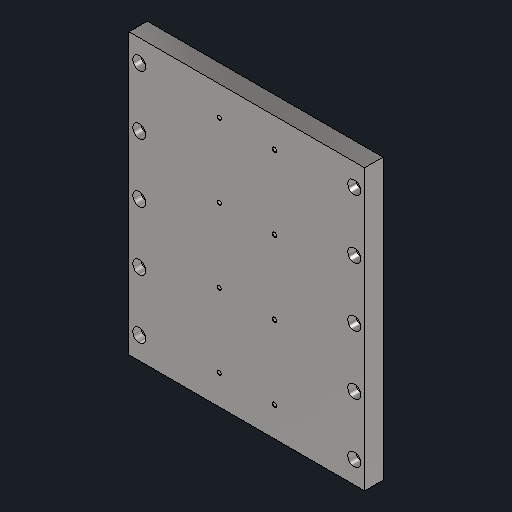
# Autodesk Inventor part: KN-00-01-03
Saved by Autodesk Inventor 2025.2 (Build 292293000, 293)
## iProperties
Created: 2025-04-28
Part Number: KN-00-01-03
Material: X5CrNi18-10
Document SubType Name: Modeling
Designer: Kacper Mik
Density: 8 g/cm^3
Appearance: Semi-Polished
Author: Kacper Mik
Autodesk Inventor part; units mm, degrees
ref_plane "YZ Plane" through (0, 0, 0) normal (1, 0, 0) x (0, 1, 0)
ref_plane "XZ Plane" through (0, 0, 0) normal (0, 1, 0) x (-1, 0, 0)
ref_plane "XY Plane" through (0, 0, 0) normal (0, 0, 1) x (1, 0, 0)
sketch "Sketch1" plane through (0, 0, 0) normal (0, 0, 1) x (1, 0, 0)
  line L0 (-160, -190) -> (160, -190)
  line L1 (160, -190) -> (160, 190)
  line L2 (160, 190) -> (-160, 190)
  line L3 (-160, 190) -> (-160, -190)
  line L4 (-160, -190) -> (160, 190) construction
  line L5 (160, -190) -> (-160, 190) construction
  point P0 (0, 0)
  dimension "d0" = 320
  dimension "d1" = 380
  constraints: 12 end point, 2 midpoint, 2 parallel, 1 horizontal, 1 perpendicular
  measures "d0" distance of L2.end L1.end
  measures "d1" distance of L1.end L0.end
extrude "Extrusion1" add sketch "Sketch1" along normal blind 25
sketch "Sketch2" plane through (0, 0, 25) normal (0, 0, 1) x (1, 0, 0)
  line L0 (-37.5, -150) -> (37.5, -150) construction
  line L1 (37.5, -150) -> (37.5, 150) construction
  line L2 (37.5, 150) -> (-37.5, 150) construction
  line L3 (-37.5, 150) -> (-37.5, -150) construction
  line L4 (-37.5, -150) -> (37.5, 150) construction
  line L5 (37.5, -150) -> (-37.5, 150) construction
  point P0 (0, 0)
  point P1 (-37.5, 50)
  point P2 (37.5, 50)
  point P3 (-37.5, -50)
  point P4 (37.5, -50)
  dimension "d4" = 75
  dimension "d5" = 300
  dimension "d6" = 100
  dimension "d7" = 100
  dimension "d8" = 100
  constraints: 12 end point, 4 coincident, 4 point on line, 2 horizontal alignment, 2 midpoint, 2 parallel, 1 horizontal, 1 perpendicular
  measures "d4" distance of L2.end L1.end
  measures "d5" distance of L1.end L0.end
  measures "d6" distance of point (-37.5, 50) point (-37.5, 150)
  measures "d7" distance of point (-37.5, -50) point (-37.5, 50)
  measures "d8" distance of point (-37.5, -150) point (-37.5, -50)
hole "Hole1" at (-37.5, 150, 25) at (37.5, 150, 25) at (-37.5, 50, 25) at (37.5, 50, 25) at (-37.5, -50, 25) at (37.5, -50, 25) at (-37.5, -150, 25) at (37.5, -150, 25) direction (0, 0, -1) diameter 5.134 end through all thread size "M6x0.8" class "6H" standard "ISO Metric profile"
chamfer "Chamfer1" distance 0.5 angle 45 8 edges at (-37.5, -147.433, 25) (-37.5, -47.433, 25) (37.5, -147.433, 25) (37.5, -47.433, 25) (-37.5, 52.567, 25) (-37.5, 152.567, 25) (37.5, 52.567, 25) (37.5, 152.567, 25)
sketch "Sketch5" plane through (0, 0, 25) normal (0, 0, 1) x (1, 0, 0)
  circle A0 centre (37.5, -150) radius 3.067 construction
  circle A1 centre (-37.5, -50) radius 3.067 construction
  circle A2 centre (-37.5, 50) radius 3.067 construction
  circle A3 centre (-37.5, 150) radius 3.067 construction
  line L0 (160, -190) -> (160, 190) construction
  line L1 (160, 190) -> (-160, 190) construction
  line L2 (-160, 190) -> (-160, -190) construction
  line L3 (-160, -190) -> (160, -190) construction
  circle A4 centre (37.5, 150) radius 3.067 construction
  circle A5 centre (37.5, 50) radius 3.067 construction
  circle A6 centre (37.5, -50) radius 3.067 construction
  circle A7 centre (-37.5, -150) radius 3.067 construction
  line L4 (146, 190) -> (146, -190) construction
  line L5 (160, -190) -> (160, 190) projected
  line L6 (160, 190) -> (-160, 190) projected
  line L7 (-160, -190) -> (160, -190) projected
  line L8 (0, 190) -> (0, -190) construction
  point P0 (0, 0)
  point P1 (146, 160)
  point P2 (146, 80)
  point P3 (146, 0)
  point P4 (146, -80)
  point P5 (146, -160)
  point P6 (-146, 160)
  point P7 (-146, 80)
  point P8 (-146, 0)
  point P9 (-146, -80)
  point P10 (-146, -160)
  dimension "d49" = 14
  dimension "d50" = 80
  dimension "d51" = 80
  dimension "d52" = 80
  dimension "d53" = 30
  dimension "d54" = 80
  dimension "d55" = 30
  constraints: 6 point on line, 5 symmetric about line, 4 end point, 3 midpoint, 1 perpendicular
  measures "d49" distance between parallel lines of L5 L4
  measures "d50" distance of point (146, 80) point (146, 160)
  measures "d51" distance of point (146, 0) point (146, 80)
  measures "d52" distance of point (146, -80) point (146, 0)
  measures "d53" distance from line of L6 point (146, 160)
  measures "d54" distance of point (146, -80) point (146, -160)
  measures "d55" distance from line of L7 point (146, -160)
hole "Hole4" at (146, 160, 25) at (146, 80, 25) at (146, 0, 25) at (146, -80, 25) at (146, -160, 25) at (-146, 160, 25) at (-146, 80, 25) at (-146, 0, 25) at (-146, -80, 25) at (-146, -160, 25) direction (0, 0, -1) diameter 10.5 end through all counterbore diameter 18 counterbore depth 11 clearance for "Socket Head Cap Screw ISO 4762" size "M10" standard "ISO"
sketch "Sketch3" plane through (160, -190, 0) normal (1, 0, 0) x (0, 0, -1)
  line L0 (0, 380) -> (-25, 380) construction
  line L1 (-12.5, 380) -> (-12.5, 0) construction
  line L2 (0, 0) -> (-25, 0) construction
  point P0 (0, 190)
  point P1 (-12.5, 315)
  point P2 (-12.5, 250)
  point P3 (-12.5, 185)
  point P4 (-12.5, 120)
  point P5 (-12.5, 55)
  dimension "d19" = 65
  dimension "d20" = 65
  dimension "d21" = 65
  dimension "d22" = 65
  dimension "d25" = 65
  dimension "d26" = 55
  constraints: 5 point on line, 2 end point, 2 midpoint
  measures "d19" distance from line of point (-12.5, 315) L0
  measures "d20" distance of point (-12.5, 250) point (-12.5, 315)
  measures "d21" distance of point (-12.5, 250) point (-12.5, 185)
  measures "d22" distance of point (-12.5, 120) point (-12.5, 185)
  measures "d25" distance of point (-12.5, 55) point (-12.5, 120)
  measures "d26" distance from line of L2 point (-12.5, 55)
sketch "Sketch4" plane through (-160, -190, 0) normal (-1, 0, 0) x (0, 0, 1)
  line L0 (0, 380) -> (25, 380) construction
  line L1 (12.5, 380) -> (12.5, 0) construction
  line L2 (0, 0) -> (25, 0) construction
  line L3 (0, 380) -> (25, 380) projected
  point P0 (0, 190)
  point P1 (12.5, 55)
  point P2 (12.5, 315)
  point P3 (12.5, 250)
  point P4 (12.5, 185)
  point P5 (12.5, 120)
  dimension "d37" = 65
  dimension "d38" = 65
  dimension "d39" = 65
  dimension "d40" = 65
  dimension "d41" = 65
  constraints: 5 point on line, 2 end point, 2 midpoint
  measures "d37" distance of point (12.5, 185) point (12.5, 120)
  measures "d38" distance of point (12.5, 250) point (12.5, 185)
  measures "d39" distance from line of L3 point (12.5, 315)
  measures "d40" distance of point (12.5, 315) point (12.5, 250)
  measures "d41" distance of point (12.5, 120) point (12.5, 55)
equation "\"d51\" = d50"
equation "\"d52\" = d50"
equation "\"d54\" = d52"
equation "\"d20\" = d19"
equation "\"d21\" = d19"
equation "\"d22\" = d19"
equation "\"d25\" = d22"
equation "\"d37\" = d38"
equation "\"d38\" = d40"
equation "\"d40\" = d39"
equation "\"d41\" = d37"
body "Solid1"
